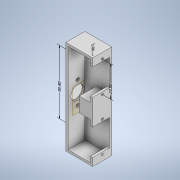
# Autodesk Inventor part: corpo
Saved by Autodesk Inventor 2022.2 (Build 262287010, 287A)
## iProperties
Created: 2021-08-02
Part Number: corpo
Material: Generic
Document SubType Name: Modeling
Designer: nakai
Density: 1 g/cm^3
Appearance: Default
Author: nakai
Autodesk Inventor part; units mm, degrees
ref_plane "YZ Plane" through (0, 0, 0) normal (1, 0, 0) x (0, 1, 0)
ref_plane "XZ Plane" through (0, 0, 0) normal (0, 1, 0) x (-1, 0, 0)
ref_plane "XY Plane" through (0, 0, 0) normal (0, 0, 1) x (1, 0, 0)
sketch "Sketch1" plane through (0, 0, 0) normal (0, 0, 1) x (1, 0, 0)
  line L0 (0, 0) -> (24, 0)
  line L1 (24, 0) -> (24, -80)
  line L2 (24, -80) -> (0, -80)
  line L3 (0, -80) -> (0, 0)
  dimension "d0" = 24
  dimension "d1" = 80
  constraints: 8 end point, 2 parallel, 1 horizontal, 1 perpendicular
  measures "d0" distance of L1.end L2.end
  measures "d1" distance of L0.end L1.end
extrude "Extrusion1" add sketch "Sketch1" along normal blind 2
sketch "Sketch2" plane through (0, 0, 2) normal (0, 0, 1) x (1, 0, 0)
  line L0 (0, -80) -> (24, -80) projected
  line L1 (0, 0) -> (2, 0)
  line L2 (2, 0) -> (2, -80)
  line L3 (2, -80) -> (0, -80)
  line L4 (0, -80) -> (0, 0)
  line L5 (24, -80) -> (24, 0) projected
  line L6 (24, 0) -> (22, 0)
  line L7 (22, 0) -> (22, -80)
  line L8 (22, -80) -> (24, -80)
  line L9 (24, -80) -> (24, 0)
  dimension "d4" = 2
  dimension "d5" = 2
  constraints: 16 end point, 4 parallel, 2 horizontal, 2 perpendicular, 2 point on line
  measures "d4" distance of L2.end L3.end
  measures "d5" distance of L8.end L7.end
extrude "Extrusion2" add sketch "Sketch2" along normal blind 15
sketch "Sketch3" plane through (24, -80, 0) normal (1, 0, 0) x (0, 0, -1)
  circle A0 centre (-8.5, 77) radius 1
  circle A1 centre (-8.5, 49.5) radius 1
  line L0 (-17, 0) -> (-17, 80) projected
  line L1 (0, 80) -> (-17, 80) projected
  dimension "d8" = 2
  dimension "d9" = 2
  dimension "d10" = 8.5
  dimension "d11" = 8.5
  dimension "d12" = 27.5
  dimension "d13" = 3
  constraints: 2 centre point
  measures "d8" diameter of A0
  measures "d9" diameter of A1
  measures "d10" distance from line of L0 A0.centre
  measures "d11" distance from line of L0 A1.centre
  measures "d12" distance of A1.centre A0.centre
  measures "d13" distance from line of L1 A0.centre
extrude "Extrusion3" cut sketch "Sketch3" against normal up to surface (2 mm away)
sketch "Sketch4" plane through (24, -80, 0) normal (1, 0, 0) x (0, 0, -1)
  line L0 (-17, 80) -> (-17, 0) projected
  line L1 (-2, 75) -> (-2, 51.5)
  circle A0 centre (-8.5, 77) radius 1 projected
  circle A1 centre (-8.5, 49.5) radius 1 projected
  line L2 (0, 0) -> (0, 80) projected
  line L3 (-2, 75) -> (-17, 75)
  line L4 (-17, 75) -> (-17, 51.5)
  line L5 (-17, 51.5) -> (-2, 51.5)
  point P0 (-17, 95)
  dimension "d24" = 23.5
  dimension "d104" = 15
  dimension "d105" = 2
  dimension "d106" = 2
  constraints: 8 end point, 2 perpendicular, 1 horizontal, 1 point on line
  measures "d24" distance of L1.start L1.end
  measures "d104" distance between parallel lines of L4 L1
  measures "d105" distance between parallel lines of L2 L1
  measures "d106" distance from line of A0.centre L3
extrude "Extrusion4" cut sketch "Sketch4" against normal up to surface (2 mm away) contours L3 L1 L5 L0
sketch "Sketch5" plane through (0, -80, 0) normal (-1, 0, 0) x (0, 0, 1)
  circle A0 centre (8.5, 68.4) radius 2.5
  circle A1 centre (8.5, 77) radius 1 projected
  point P0 (0, 80)
  dimension "d29" = 5
  dimension "d32" = 8.6
  dimension "d33" = 0
  constraints: 1 centre point
  measures "d29" diameter of A0
  measures "d32" distance of A1.centre A0.centre
  measures "d33" horizontal distance of A0.centre A1.centre
extrude "Extrusion5" add sketch "Sketch5" along normal blind 5 contours A0
sketch "Sketch15" plane through (0, 0, 0) normal (0, 1, 0) x (1, 0, 0)
  line L0 (22, -17) -> (24, -17) projected
  line L1 (0, 0) -> (0, -17) projected
  line L2 (24, -17) -> (0, -17)
  line L3 (0, -17) -> (0, 0)
  line L4 (0, 0) -> (24, 0)
  line L5 (24, 0) -> (24, -17)
  point P0 (22, -17)
  constraints: 8 end point, 2 parallel, 1 horizontal, 1 perpendicular
extrude "Extrusion12" add sketch "Sketch15" along normal blind 2
sketch "Sketch16" plane through (24, -80, 17) normal (1, 0, 0) x (0, 0, -1)
  line L0 (0, 80) -> (0, 0) projected
  line L1 (0, 5) -> (15, 5)
  line L2 (15, 5) -> (15, 28.5)
  line L3 (15, 28.5) -> (0, 28.5)
  line L4 (0, 28.5) -> (0, 5)
  line L5 (17, 0) -> (0, 0) projected
  circle A0 centre (8.5, 3) radius 1
  circle A1 centre (8.5, 30.5) radius 1
  point P0 (17, 80)
  point P1 (0, 71.5)
  point P2 (7.5, 5)
  point P3 (7.5, 28.5)
  point P4 (0, 28.5)
  dimension "d84" = 15
  dimension "d85" = 23.5
  dimension "d86" = 5
  dimension "d87" = 2
  dimension "d88" = 2
  dimension "d89" = 8.5
  dimension "d90" = 8.5
  dimension "d91" = 2
  dimension "d92" = 2
  constraints: 8 end point, 2 centre point, 2 midpoint, 2 parallel, 1 horizontal, 1 perpendicular, 1 point on line
  measures "d84" distance of L3.end L2.end
  measures "d85" distance of L2.end L1.end
  measures "d86" distance between parallel lines of L5 L1
  measures "d87" diameter of A0
  measures "d88" diameter of A1
  measures "d89" distance from line of L0 A1.centre
  measures "d90" distance from line of L0 A0.centre
  measures "d91" vertical distance of point (7.5, 5) A0.centre
  measures "d92" vertical distance of A1.centre point (7.5, 28.5)
extrude "Extrusion13" cut sketch "Sketch16" against normal up to surface (2 mm away)
sketch "Sketch17" plane through (0, -80, 0) normal (0, -1, 0) x (1, 0, 0)
  line L0 (24, 4) -> (24, 17) projected
  line L1 (24, 17) -> (0, 17)
  line L2 (0, 17) -> (0, 0)
  line L3 (0, 0) -> (24, 0)
  line L4 (24, 0) -> (24, 17)
  point P0 (24, 2)
  constraints: 8 end point, 2 parallel, 1 horizontal, 1 perpendicular
extrude "Extrusion14" add sketch "Sketch17" along normal blind 2
sketch "Sketch18" plane through (0, 2, 0) normal (-1, 0, 0) x (0, 0, 1)
  circle A0 centre (8.5, -70.4) radius 2.5
  line L0 (17, -84) -> (0, -84) projected
  line L1 (17, -84) -> (17, 0) projected
  point P0 (0, -2)
  dimension "d97" = 5
  dimension "d98" = 13.6
  dimension "d99" = 8.5
  constraints: 1 centre point
  measures "d97" diameter of A0
  measures "d98" distance from line of L0 A0.centre
  measures "d99" distance from line of L1 A0.centre
extrude "Extrusion15" add sketch "Sketch18" along normal blind 5
ref_plane "Plano de trabalho3" through (2, -44.5, 2) normal (1, 0, 0) x (0, 0, -1)
sketch "Sketch21" plane through (2, -44.5, 2) normal (1, 0, 0) x (0, 0, -1)
  circle A0 centre (-6.5, 4.5) radius 6
  line L0 (0, 9) -> (-15, 9) projected
  line L1 (-15, -35.5) -> (-15, 44.5) projected
  circle A1 centre (-6.4973, 14.5) radius 1.5
  circle A2 centre (-6.5, -5.5) radius 1.5
  line L2 (0, 44.5) -> (-15, 44.5) projected
  point P0 (2, 44.5)
  point P1 (-15, 0)
  point P2 (-15, 46.5)
  dimension "d122" = 12
  dimension "d124" = 8.5
  dimension "d129" = 3
  dimension "d130" = 3
  dimension "d131" = 10
  dimension "d132" = 10
  dimension "d134" = 40
  constraints: 3 centre point
  measures "d122" diameter of A0
  measures "d124" distance from line of L1 A0.centre
  measures "d129" diameter of A1
  measures "d130" diameter of A2
  measures "d131" distance of A1.centre A0.centre
  measures "d132" distance of A0.centre A2.centre
  measures "d134" distance from line of L2 A0.centre
extrude "Extrusion18" cut sketch "Sketch21" against normal up to surface (2 mm away)
sketch "Esboço22" plane through (0, 0, 2) normal (0, 0, 1) x (1, 0, 0)
  line L0 (22, -51.5) -> (22, -28.5) projected
  line L1 (22, -33.5) -> (12, -33.5)
  line L2 (12, -33.5) -> (12, -46.5)
  line L3 (12, -46.5) -> (22, -46.5)
  line L4 (22, -46.5) -> (22, -33.5)
  line L5 (24, -28.5) -> (22, -28.5) projected
  line L6 (22, -51.5) -> (24, -51.5) projected
  point P0 (0, 0)
  dimension "d142" = 10
  dimension "d143" = 5
  dimension "d144" = 5
  constraints: 8 end point, 2 parallel, 1 horizontal, 1 perpendicular, 1 point on line
  measures "d142" distance of L3.end L2.end
  measures "d143" distance between parallel lines of L5 L1
  measures "d144" distance between parallel lines of L6 L3
extrude "Extrusão19" add sketch "Esboço22" along normal up to surface (15 mm away)
equation "\"d11\" = d10"
equation "\"d90\" = d89"
body "Solid1"
